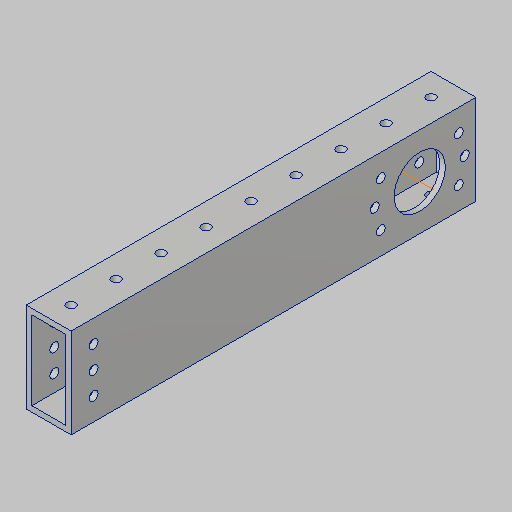
# Autodesk Inventor part: CL3-001
Saved by Autodesk Inventor 2023.5 (Build 275446000, 446)
## iProperties
RuleStatus: InUse
Created: 2025-01-28
Part Number: CL3-001
Material: Aluminum 6061
Document SubType Name: Modeling
Designer: slick
Mass: 304.185 g
Surface Area: 718.547 cm^2
Volume: 112.661 cm^3
Density: 2.7 g/cm^3
Appearance: Aluminum - Flat
AfterDocNew0: SHOW
AfterDocOpen0: SHOW
Author: slick
Autodesk Inventor part; units mm, degrees
ref_plane "YZ Plane" through (0, 0, 0) normal (1, 0, 0) x (0, 1, 0)
ref_plane "XZ Plane" through (0, 0, 0) normal (0, 1, 0) x (-1, 0, 0)
ref_plane "XY Plane" through (0, 0, 0) normal (0, 0, 1) x (1, 0, 0)
sketch "Sketch1" plane through (0, 0, 0) normal (0, 0, 1) x (1, 0, 0)
  line L0 (-12.7, -25.4) -> (12.7, -25.4)
  line L1 (12.7, -25.4) -> (12.7, 25.4)
  line L2 (12.7, 25.4) -> (-12.7, 25.4)
  line L3 (-12.7, 25.4) -> (-12.7, -25.4)
  line L4 (-12.7, -25.4) -> (12.7, 25.4) construction
  line L5 (12.7, -25.4) -> (-12.7, 25.4) construction
  line L6 (-9.525, 22.225) -> (9.525, 22.225)
  line L7 (9.525, 22.225) -> (9.525, -22.225)
  line L8 (9.525, -22.225) -> (-9.525, -22.225)
  line L9 (-9.525, -22.225) -> (-9.525, 22.225)
  point P0 (0, 0)
  dimension "width" = 25.4
  dimension "height" = 50.8
  dimension "thickness" = 3.175
  constraints: 20 end point, 4 parallel, 2 midpoint, 2 perpendicular, 1 horizontal, 3 other
  measures "width" distance of L2.end L1.end
  measures "height" distance of L1.end L0.end
  measures "thickness" distance between parallel lines of L2 L6
extrude "Extrusion1" add sketch "Sketch1" along normal mid plane 228.6
sketch "Sketch3" plane through (-12.7, -25.4, -114.3) normal (-1, 0, 0) x (0, 0, 1)
  circle A0 centre (25.4, 25.4) radius 14.2875
  line L0 (0, 0) -> (0, 50.8) projected
  point P0 (114.3, 25.4)
  dimension "d8" = 28.575
  dimension "d9" = 25.4
  constraints: 1 centre point, 1 horizontal alignment
  measures "d8" diameter of A0
  measures "d9" distance from line of L0 A0.centre
extrude "Extrusion3" [suppressed]
sketch "Sketch4" plane through (-12.7, 25.4, 114.3) normal (0, 1, 0) x (1, 0, 0)
  line L0 (0, 228.6) -> (0, 0) projected
  line L1 (25.4, 0) -> (0, 0) projected
  line L2 (25.4, 228.6) -> (25.4, 0) projected
  line L3 (0, 228.6) -> (25.4, 228.6) construction
  line L4 (0, 228.6) -> (0, 0) construction
  line L5 (25.4, 228.6) -> (25.4, 0) construction
  line L6 (0, 0) -> (25.4, 0) construction
  line L7 (25.4, 0) -> (0, 25.4)
  line L8 (0, 25.4) -> (0, 0)
  line L9 (0, 0) -> (25.4, 0)
  point P0 (12.7, 114.3)
  point P1 (0, 25.4)
  dimension "d17" = 45
  constraints: 6 end point, 2 collinear, 1 point on line
  measures "d17" angle of L1 L7
extrude "Extrusion4" [suppressed]
sketch "Sketch5" plane through (-12.7, 25.4, -114.3) normal (0, 1, 0) x (1, 0, 0)
  line L0 (0, 0) -> (25.4, 0) construction
  line L1 (25.4, 0) -> (25.4, -228.6) construction
  line L2 (0, -228.6) -> (0, 0) construction
  line L3 (25.4, -228.6) -> (0, -228.6) projected
  point P0 (12.7, -114.3)
  point P1 (12.7, -12.7)
  point P2 (12.7, 0)
  dimension "d18" = 12.7
  constraints: 1 midpoint, 1 vertical alignment
  measures "d18" distance from line of L0 point (12.7, -12.7)
hole "Hole1" at (0, 25.4, -101.6) direction (0, -1, 0) diameter 5.1054 end through all clearance for "Flat Head Machine Screw (82)" size "#10" standard "Ansi Unified Screw Threads"
pattern_linear "Rectangular Pattern1" count 9 spacing 25.4 along (0, 0, 1) of "Hole1"
sketch "Sketch6" plane through (-12.7, 25.4, 114.3) normal (0, 1, 0) x (1, 0, 0)
  circle A0 centre (12.7, 38.1) radius 2.5527 construction
  circle A1 centre (12.7, 63.5) radius 2.5527 construction
  circle A2 centre (12.7, 88.9) radius 2.5527 construction
  circle A3 centre (12.7, 114.3) radius 2.5527 construction
  circle A4 centre (12.7, 139.7) radius 2.5527 construction
  circle A5 centre (12.7, 165.1) radius 2.5527 construction
  circle A6 centre (12.7, 190.5) radius 2.5527 construction
  circle A7 centre (12.7, 215.9) radius 2.5527 construction
  line L0 (0, 228.6) -> (25.4, 228.6) construction
  line L1 (25.4, 228.6) -> (25.4, 0) construction
  line L2 (25.4, 0) -> (0, 0) construction
  line L3 (0, 0) -> (0, 228.6) construction
  line L4 (25.4, 0) -> (25.4, 25.4)
  line L5 (25.4, 25.4) -> (0, 0)
  line L6 (0, 0) -> (25.4, 0)
  circle A8 centre (12.7, 12.7) radius 2.5527 projected
  dimension "d29" = 45
  constraints: 6 end point, 1 vertical
  measures "d29" angle of L2 L5
extrude "Extrusion5" [suppressed]
sketch "Sketch7" plane through (12.7, -25.4, 114.3) normal (1, 0, 0) x (0, 0, -1)
  line L0 (228.6, 50.8) -> (228.6, 0) construction
  line L1 (228.6, 0) -> (0, 0) construction
  line L2 (0, 0) -> (0, 50.8) construction
  line L3 (0, 50.8) -> (228.6, 50.8) construction
  point P0 (114.3, 25.4)
  point P1 (12.7, 38.1)
  point P2 (12.7, 25.4)
  point P3 (12.7, 12.7)
  point P4 (0, 25.4)
  dimension "d32" = 12.7
  dimension "d33" = 12.7
  dimension "d34" = 12.7
  constraints: 2 vertical alignment, 1 horizontal alignment, 1 midpoint
  measures "d32" distance of point (12.7, 25.4) point (12.7, 38.1)
  measures "d33" distance of point (12.7, 12.7) point (12.7, 25.4)
  measures "d34" distance from line of L2 point (12.7, 25.4)
hole "Hole2" at (12.7, 12.7, 101.6) at (12.7, 0, 101.6) at (12.7, -12.7, 101.6) direction (-1, 0, 0) diameter 5.1054 end through all clearance for "Flat Head Machine Screw (82)" size "#10" standard "Ansi Unified Screw Threads"
sketch "Sketch8" plane through (12.7, -25.4, 114.3) normal (1, 0, 0) x (0, 0, -1)
  circle A0 centre (12.7, 25.4) radius 2.5527 construction
  circle A1 centre (12.7, 38.1) radius 2.5527 construction
  circle A2 centre (12.7, 12.7) radius 2.5527 construction
  line L0 (228.6, 50.8) -> (228.6, 0) construction
  line L1 (228.6, 0) -> (0, 0) construction
  line L2 (0, 0) -> (0, 50.8) construction
  line L3 (0, 50.8) -> (228.6, 50.8) construction
  circle A3 centre (196.85, 25.4) radius 23.8125 construction
  circle A4 centre (196.85, 25.4) radius 25.4 construction
  circle A5 centre (196.85, 25.4) radius 50.8 construction
  circle A6 centre (196.85, 25.4) radius 76.2 construction
  point P0 (114.3, 25.4)
  point P1 (220.6625, 25.4)
  point P2 (218.847, 38.1)
  point P3 (208.7562, 46.0222)
  point P4 (184.9437, 46.0222)
  point P5 (173.0375, 25.4)
  point P6 (184.9437, 4.7778)
  point P7 (208.7562, 4.7778)
  point P8 (209.55, 47.397)
  point P9 (196.85, 50.8)
  point P10 (184.15, 47.397)
  point P11 (174.853, 38.1)
  point P12 (171.45, 25.4)
  point P13 (174.853, 12.7)
  point P14 (184.15, 3.403)
  point P15 (196.85, 0)
  point P16 (209.55, 3.403)
  point P17 (218.847, 12.7)
  point P18 (222.25, 25.4)
  dimension "d42" = 47.625
  dimension "d43" = 50.8
  dimension "d44" = 101.6
  dimension "d45" = 152.4
  dimension "d46" = 31.75
  dimension "d49" = 360
  dimension "d53" = 360
  constraints: 3 coincident, 3 horizontal alignment, 2 centre point, 1 vertical alignment, 25 other
  measures "d44" diameter of A5
  measures "d45" diameter of A6
  measures "d46" distance from line of L0 point (196.85, 25.4)
hole "Hole3" [suppressed]
hole "Hole4" at (12.7, 12.7, -104.547) at (12.7, 12.7, -60.553) at (12.7, 0, -57.15) at (12.7, -12.7, -60.553) at (12.7, -12.7, -104.547) at (12.7, 0, -107.95) direction (-1, 0, 0) diameter 5.1054 end through all clearance for "Flat Head Machine Screw (82)" size "#10" standard "Ansi Unified Screw Threads"
hole "Hole5" at (12.7, 0, -82.55) direction (-1, 0, 0) diameter 28.956 end through all
equation "\"d33\" = d32"
body "Solid1"
